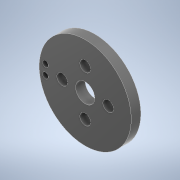
# Autodesk Inventor part: Faden_Halter_24_Durchmesser
Saved by Autodesk Inventor 2021 (Build 250183000, 183)
## iProperties
Created: 2021-05-20
Part Number: Faden_Halter_24_Durchmesser
Material: Generisch
Document SubType Name: Modeling
Designer: Maxim
Density: 1 g/cm^3
Appearance: Glatt - Schwarz
Author: Maxim
## iProperties of the stored document _3D-Druck.ipt
Created: 2021-06-11
Part Number: _3D-Druck
Material: Generisch
Document SubType Name: Modeling
Designer: Maxim
Density: 1 g/cm^3
Appearance: Vorgabe
Author: Maxim
Autodesk Inventor part; units mm, degrees
ref_plane "YZ Plane" through (0, 0, 0) normal (1, 0, 0) x (0, 1, 0)
ref_plane "XZ Plane" through (0, 0, 0) normal (0, 1, 0) x (-1, 0, 0)
ref_plane "XY Plane" through (0, 0, 0) normal (0, 0, 1) x (1, 0, 0)
sketch "Skizze1" plane through (0, 0, 0) normal (0, 0, 1) x (1, 0, 0)
  circle A0 centre (0, 0) radius 12
  circle A1 centre (0, 0) radius 2.5
  dimension "d0" = 24
  dimension "d1" = 5
  constraints: 2 centre point, 2 coincident
  measures "d0" diameter of A0
  measures "d1" diameter of A1
extrude "Extrusion1" add sketch "Skizze1" along normal blind 2.5
sketch "Skizze2" plane through (0, 0, 0) normal (0, 0, 1) x (1, 0, 0)
  circle A0 centre (-10.4, -1.3) radius 0.75
  circle A1 centre (-10.4, 1.3) radius 0.75
  line L0 (-13.98, 0) -> (2.33, 0) projected
  line L1 (0, 2.87) -> (0, -2.87) projected
  point P0 (0, 0)
  dimension "d4" = 1.5
  dimension "d5" = 1.5
  dimension "d6" = 1.3
  dimension "d7" = 1.3
  dimension "d8" = 10.4
  dimension "d9" = 10.4
  constraints: 2 centre point
  measures "d4" diameter of A0
  measures "d5" diameter of A1
  measures "d6" distance from line of L0 A0.centre
  measures "d7" distance from line of L0 A1.centre
  measures "d8" distance from line of L1 A1.centre
  measures "d9" distance from line of L1 A0.centre
extrude "Extrusion2" cut sketch "Skizze2" along normal blind 6.75
sketch "Skizze3" plane through (0, 0, 0) normal (0, 0, -1) x (-1, 0, 0)
  circle A0 centre (0, 6) radius 1.4
  line L0 (-16.8, 0) -> (16.8, 0) projected
  line L1 (0, -16.8) -> (0, 16.8) projected
  circle A1 centre (-6, 0) radius 1.4
  circle A2 centre (0, -6) radius 1.4
  circle A3 centre (6, 0) radius 1.4
  point P0 (0, 0)
  point P1 (7.4, 0)
  point P2 (4.6, 0)
  point P3 (-4.6, 0)
  point P4 (-7.4, 0)
  point P5 (0, -4.6)
  point P6 (0, -7.4)
  point P7 (0, 4.6)
  point P8 (0, 7.4)
  dimension "d12" = 2.8
  dimension "d13" = 6
  dimension "d14" = 0
  dimension "d20" = 360
  constraints: 4 centre point, 9 other
  measures "d12" diameter of A0
  measures "d13" distance from line of L0 A0.centre
  measures "d14" distance from line of L1 A0.centre
extrude "Extrusion3" cut sketch "Skizze3" against normal blind 6.75
